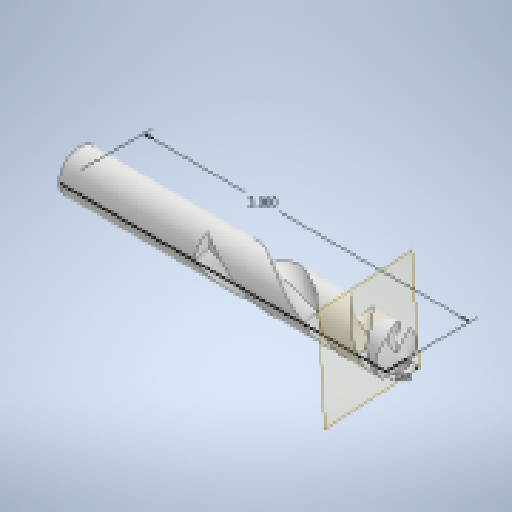
# Autodesk Inventor part: Drill_Bit
Saved by Autodesk Inventor 2023 (Build 270158000, 158)
## iProperties
Created: 2022-05-09
Part Number: Drill_Bit
Material: Generic
Document SubType Name: Modeling
Designer: plebbb
Density: 1 g/cm^3
Appearance: Default
Author: plebbb
Autodesk Inventor part; units mm, degrees
ref_plane "YZ Plane" through (0, 0, 0) normal (1, 0, 0) x (0, 1, 0)
ref_plane "XZ Plane" through (0, 0, 0) normal (0, 1, 0) x (-1, 0, 0)
ref_plane "XY Plane" through (0, 0, 0) normal (0, 0, 1) x (1, 0, 0)
sketch "Sketch1" plane through (0, 0, 0) normal (0, 1, 0) x (-1, 0, 0)
  line L0 (0, 0) -> (76.2, 0)
  line L1 (76.2, 0) -> (76.2, -4.7625)
  line L2 (76.2, -4.7625) -> (0, -4.7625)
  line L3 (0, -4.7625) -> (0, 0)
  dimension "d0" = 76.2
  dimension "d1" = 4.7625
  constraints: 8 end point, 2 parallel, 1 horizontal, 1 perpendicular
  measures "d0" distance of L1.end L2.end
  measures "d1" distance of L2.end L0.start
revolve "Revolution1" add sketch "Sketch1" angle 360 about axis through (-76.2, 0, -4.7625) along (1, 0, 0)
sketch "Sketch4" plane through (0, 0, -4.7625) normal (1, 0, 0) x (0, 0, -1)
  arc A0 (-1.56226, 0.894228) -> (-4.7625, 0) centre (3.658544, -23.963431) ccw
  circle A1 centre (0, 0) radius 4.7625
  arc A2 (-1.56226, 0.894228) -> (-1.719653, 4.441194) centre (-4.875355, 2.524188) ccw
  dimension "d33" = 25.4
  dimension "d35" = 3.69234
  dimension "d36" = 4.44119
  constraints: 5 point on circle, 2 centre point, 1 other
  measures "d33" radius of A0
  measures "d35" radius of A2
  measures "d36" vertical distance of A0.end A1.end
sketch "Sketch4 outline for Coil1" plane through (0, 0, -4.7625) normal (1, 0, 0) x (0, 0, -1)
  arc A0 (-1.719653, 4.441194) -> (-4.7625, 0) centre (0, 0) ccw
  arc A1 (-1.56226, 0.894228) -> (-1.719653, 4.441194) centre (-4.875355, 2.524188) ccw
  arc A2 (-4.7625, 0) -> (-1.56226, 0.894228) centre (3.658544, -23.963431) cw
coil "Coil1" sketch "Sketch4 outline for Coil1" operation cut axis through (-76.2, 0, -4.7625) along (-1, 0, 0) pitch 12.7 turns 0.5 hand right
ref_plane "Work Plane1" through (-6.35, 0, -4.7625) normal (1, 0, 0) x (0, 0.0653273, -0.9978639)
sketch "Sketch5" plane through (-6.35, 0, -4.7625) normal (1, 0, 0) x (0, 0.0653273, -0.9978639)
  arc A0 (1.500505, -0.994376) -> (4.752327, -0.311121) centre (-2.085262, 24.151245) ccw
  arc A1 (1.500505, -0.994376) -> (1.425848, -4.544047) centre (4.700042, -2.83729) ccw
  arc A2 (1.425848, -4.544047) -> (4.752327, -0.311121) centre (0, 0) ccw
coil "Coil2" sketch "Sketch5" operation cut axis through (-76.2, 0, -4.7625) along (-1, 0, 0) pitch 25.4 turns 0.5 hand right
sketch "Sketch6" plane through (-19.05, 0, -4.7625) normal (1, 0, 0) x (0, -0.8249491, 0.5652071)
  arc A0 (-2.691799, -3.92882) -> (2.691799, -3.92882) centre (0, 0) ccw
  arc A1 (0.145308, -1.794209) -> (2.691799, -3.92882) centre (17.700776, 16.562413) ccw
  arc A2 (0.145308, -1.794209) -> (-2.691799, -3.92882) centre (0.673259, -5.448608) ccw
  point P0 (-4.752327, 0.311121)
coil "Coil3" sketch "Sketch6" operation cut axis through (-76.2, 0, -4.7625) along (-1, 0, 0) pitch 50.8 turns 0.5 hand right
pattern_circular "Circular Pattern2" count 2 over 360 about axis through (-38.1, 0, -4.7625) along (1, 0, 0) of "Coil3", "Coil2", "Coil1"
sketch "Sketch8" plane through (0, 0, 0) normal (0, 1, 0) x (-1, 0, 0)
  line L0 (0, -4.7625) -> (0, 0)
  line L1 (0, 0) -> (2.22079, 0)
  line L2 (2.22079, 0) -> (0, -4.7625)
  dimension "d40" = 4.7625
  dimension "d41" = 25
  constraints: 6 end point, 1 coincident, 1 perpendicular, 1 vertical
  measures "d40" distance of L0.start L0.end
  measures "d41" angle of L0 L2
revolve "Revolution3" cut sketch "Sketch8" angle 360 about axis through (-76.2, 0, -4.7625) along (1, 0, 0)
body "Solid1"
